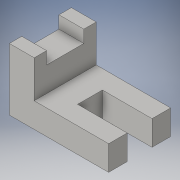
# Autodesk Inventor part: Figure 7_27_1
Saved by Autodesk Inventor 2016 (Build 200138000, 138)
## iProperties
Created: 2016-07-18
Part Number: Figure 7_27_1
Material: Generic
Document SubType Name: Modeling
Designer: cfkguest
Density: 1 g/cm^3
Appearance: Default
Author: cfkguest
Autodesk Inventor part; units mm, degrees
ref_plane "YZ Plane" through (0, 0, 0) normal (1, 0, 0) x (0, 1, 0)
ref_plane "XZ Plane" through (0, 0, 0) normal (0, 1, 0) x (-1, 0, 0)
ref_plane "XY Plane" through (0, 0, 0) normal (0, 0, 1) x (1, 0, 0)
sketch "Sketch1" plane through (0, 0, 0) normal (0, 0, 1) x (1, 0, 0)
  line L0 (-19.8053, 20.7004) -> (-19.8053, -11.0496)
  line L1 (-19.8053, -11.0496) -> (30.9947, -11.0496)
  line L2 (30.9947, -11.0496) -> (30.9947, 1.6504)
  line L3 (30.9947, 1.6504) -> (-7.1053, 1.6504)
  line L4 (-7.1053, 1.6504) -> (-7.1053, 20.7004)
  line L5 (-7.1053, 20.7004) -> (-19.8053, 20.7004)
  point P0 (0, 0)
  dimension "d0" = 12.7
  dimension "d1" = 50.8
  dimension "d2" = 12.7
  dimension "d3" = 31.75
  constraints: 12 end point, 5 perpendicular, 1 vertical
  measures "d0" distance of L4.end L0.start
  measures "d1" distance of L0.end L1.end
  measures "d2" distance of L1.end L2.end
  measures "d3" distance of L0.start L0.end
extrude "Extrusion1" add sketch "Sketch1" along normal blind 31.75
sketch "Sketch2" plane through (-7.1053, 1.6504, 0) normal (1, 0, 0) x (0, 0, -1)
  line L0 (0, 19.05) -> (-31.75, 19.05) projected
  line L1 (-25.4, 19.05) -> (-6.35, 19.05)
  line L2 (-6.35, 19.05) -> (-6.35, 12.7)
  line L3 (-6.35, 12.7) -> (-25.4, 12.7)
  line L4 (-25.4, 12.7) -> (-25.4, 19.05)
  line L5 (-31.75, 0) -> (-31.75, 19.05) projected
  line L6 (0, 0) -> (0, 19.05) projected
  point P0 (0, -1.6504)
  dimension "d6" = 6.35
  dimension "d7" = 6.35
  dimension "d8" = 6.35
  constraints: 8 end point, 2 parallel, 1 horizontal, 1 perpendicular, 1 point on line
  measures "d6" distance between parallel lines of L5 L4
  measures "d7" distance between parallel lines of L2 L6
  measures "d8" distance of L3.end L1.start
extrude "Extrusion2" cut sketch "Sketch2" against normal blind 31.75
sketch "Sketch3" plane through (-7.1053, 1.6504, 0) normal (0, 1, 0) x (1, 0, 0)
  line L0 (38.1, 0) -> (38.1, -31.75) projected
  line L1 (38.1, -22.225) -> (12.7, -22.225)
  line L2 (12.7, -22.225) -> (12.7, -9.525)
  line L3 (12.7, -9.525) -> (38.1, -9.525)
  line L4 (38.1, -9.525) -> (38.1, -22.225)
  line L5 (-12.7, 0) -> (38.1, 0) projected
  line L6 (38.1, -31.75) -> (0, -31.75) projected
  point P0 (7.1053, 0)
  dimension "d11" = 9.525
  dimension "d12" = 9.525
  dimension "d13" = 25.4
  constraints: 8 end point, 2 parallel, 1 horizontal, 1 perpendicular, 1 point on line
  measures "d11" distance between parallel lines of L5 L3
  measures "d12" distance between parallel lines of L6 L1
  measures "d13" distance of L1.start L1.end
extrude "Extrusion3" cut sketch "Sketch3" against normal blind 31.75
body "Solid1"
